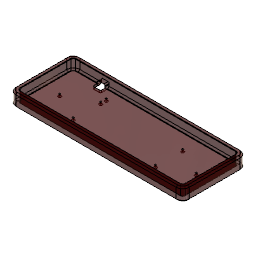
PlanckHiProCase (Autodesk Fusion 360 design; units mm, degrees)
part number: 2025-12-26-20-35-43-522
Autodesk Fusion 360 part; units mm, degrees
ref_plane "WorkPlane1" through (0, 0, -6) normal (0, 0, 1) x (1, 0, 0)
ref_plane "WorkPlane2" through (0, 0, -5) normal (0, 0, 1) x (1, 0, 0)
other "Base Mesh Feature2"
sketch "Floor" plane through (0, 0, -5) normal (0, 0, 1) x (1, 0, 0)
  circle A0 centre (-95, -0.0001) radius 1.0986
  circle A1 centre (-56.999, 27.0014) radius 0.9987
  circle A2 centre (-57, 18.9999) radius 1.0986
  circle A3 centre (-57, -19) radius 1.0985
  circle A4 centre (57, -19) radius 1.0985
  circle A5 centre (57, 18.9999) radius 1.0986
  circle A6 centre (95, -0.0001) radius 1.0986
  line L0 (-81.249, 50.7868) -> (-81.249, 32.4014)
  line L1 (-81.249, 32.4014) -> (-70.749, 32.4014)
  line L2 (-70.749, 32.4014) -> (-70.749, 50.7879)
  line L3 (-81.249, 50.7868) -> (-70.749, 50.7879)
  dimension "d10" = 10.5
  dimension "d21" = 5.4
  dimension "d22" = 13.75
  constraint horizontal L1
  constraint vertical L0
  constraint vertical L2
  constraint coincident L0.end L1.start
  constraint coincident L1.end L2.start
  measures "d10" distance of L0 L2
  measures "d21" distance of A1.centre L1
  measures "d22" distance of A1.centre L2
other "MeshSection1"
sketch "Walls" plane through (0, 0, -6) normal (0, 0, 1) x (1, 0, 0)
  line L0 (111.325, 38.5) -> (-111.325, 38.5)
  arc A0 (114.5, 35.325) -> (111.325, 38.5) centre (111.325, 35.325) ccw
  line L1 (114.5, -35.325) -> (114.5, 35.325)
  arc A1 (111.325, -38.5) -> (114.5, -35.325) centre (111.325, -35.325) ccw
  line L2 (-111.325, -38.5) -> (111.325, -38.5)
  arc A2 (-114.5, -35.325) -> (-111.325, -38.5) centre (-111.325, -35.325) ccw
  line L3 (-114.5, 35.325) -> (-114.5, -35.325)
  arc A3 (-111.325, 38.5) -> (-114.5, 35.325) centre (-111.325, 35.325) ccw
  line L4 (-120.5, 35.325) -> (-120.5, -35.325)
  arc A4 (-120.5, -35.325) -> (-111.325, -44.5) centre (-111.325, -35.325) ccw
  line L5 (-111.325, -44.5) -> (111.325, -44.5)
  arc A5 (111.325, -44.5) -> (120.5, -35.325) centre (111.325, -35.325) ccw
  line L6 (120.5, -35.325) -> (120.5, 35.325)
  arc A6 (120.5, 35.325) -> (111.325, 44.5) centre (111.325, 35.325) ccw
  line L7 (111.325, 44.5) -> (-111.325, 44.5)
  arc A7 (-111.325, 44.5) -> (-120.5, 35.325) centre (-111.325, 35.325) ccw
  dimension "d23" = 38.5
  dimension "d24" = 38.5
  dimension "d25" = 114.5
  dimension "d26" = 114.5
  dimension "d28" = 3.175
  dimension "d29" = 6
  constraint horizontal L2
  constraint horizontal L0
  constraint tangent L2 A2
  constraint tangent A1 L2
  constraint tangent L0 A0
  constraint tangent L0 A3
  constraint tangent A2 L3
  constraint vertical L3
  constraint vertical L1
  constraint tangent L1 A1
  constraint tangent A0 L1
  constraint tangent L3 A3
  constraint coincident L3.start A3.end
  constraint equal A2 A3
  constraint equal A1 A3
  constraint equal A0 A3
  measures "d23" distance of origin L0
  measures "d24" distance of origin L2
  measures "d25" distance of origin L3
  measures "d26" distance of origin L1
  measures "d28" radius of A3
other "MeshSection2"
ref_plane "WorkPlane3" through (0, 38.5, 0) normal (0, 1, 0) x (0, 0, 1)
sketch "BackCutout" plane through (0, 38.5, 0) normal (0, 1, 0) x (-1, 0, 0)
  line L0 (70.75, -1.9309) -> (70.75, -14.816)
  line L1 (81.25, -1.9309) -> (70.75, -1.9309)
  line L2 (70.75, -14.816) -> (81.25, -14.816)
  line L3 (115.5, -9.0707) -> (70.75, -9.0709) construction
  line L4 (-115.5, -9.0698) -> (70.75, -9.0709) construction
  line L5 (81.25, -1.9309) -> (81.25, -14.816)
  point P0 (76, -1.9309)
  dimension "d37" = 7.14
  dimension "d39" = 5.25
  dimension "d40" = 5.25
  constraint horizontal L1
  constraint vertical L0
  constraint midpoint L1 P0
  constraint horizontal L2
  constraint vertical L5
  constraint coincident L1.start L5.start
  constraint coincident L0.start L1.end
  measures "d37" distance of P0 L3
  measures "d39" distance of P0 L5
  measures "d40" distance of L0 P0
other "MeshSection3"
extrude "Extrude1" add sketch "Walls" against normal blind 3 contours L0 A0 L1 A1 L2 A2 L3 A3 | L4 A4 L5 A5 L6 A6 L7 A7
extrude "Extrude2" add sketch "Walls" along normal blind 15
extrude "CutDown" cut sketch "Floor" against normal through all contours L0 L1 L2 L3
extrude "CutBack" cut sketch "BackCutout" along normal through all
chamfer "Chamfer1" distance 0.5 angle 45 8 edges at (-113.5701, 37.5701, 9) (0, 38.5, 9) (113.5701, 37.5701, 9) (114.5, 0, 9) (113.5701, -37.5701, 9) (0, -38.5, 9) (-113.5701, -37.5701, 9) (-114.5, 0, 9)
chamfer "Chamfer1" distance 2 angle 45 8 edges at (-120.5, 0, 9) (-117.8127, -41.8127, 9) (0, -44.5, 9) (117.8127, -41.8127, 9) (120.5, 0, 9) (117.8127, 41.8127, 9) (0, 44.5, 9) (-117.8127, 41.8127, 9)
chamfer "Chamfer1" distance 2 angle 45 9 edges at (-96.287, 44.5, -9) (20.288, 44.5, -9) (117.8127, 41.8127, -9) (120.5, 0, -9) (117.8127, -41.8127, -9) (0, -44.5, -9) (-117.8127, -41.8127, -9) (-120.5, 0, -9) (-117.8127, 41.8127, -9)
fillet "Fillet2" radius 1.5875 2 edges at (-81.249, 32.4014, -7.5) (-70.749, 32.4014, -7.5)
fillet "Fillet2" radius 1.5875 2 edges at (-81.25, 41.5, -1.9309) (-70.75, 41.5, -1.9309)
sketch "Holes" plane through (0, 0, -9) normal (0, 0, -1) x (1, 0, 0)
  line L0 (-81.249, -38.5) -> (-81.249, -33.9889)
  line L1 (-79.6615, -32.4014) -> (-72.3365, -32.4014)
  line L2 (-70.749, -33.9889) -> (-70.749, -42.5)
  line L3 (-81.25, -38.5) -> (-81.249, -38.5)
  line L4 (-81.25, -42.5) -> (-81.25, -38.5)
  arc A0 (-79.6615, -32.4014) -> (-81.249, -33.9889) centre (-79.6615, -33.9889) ccw
  arc A1 (-70.749, -33.9889) -> (-72.3365, -32.4014) centre (-72.3365, -33.9889) ccw
  line L5 (-70.749, -42.5) -> (111.325, -42.5)
  arc A2 (111.325, -42.5) -> (118.5, -35.325) centre (111.325, -35.325) ccw
  line L6 (118.5, -35.325) -> (118.5, 35.325)
  arc A3 (118.5, 35.325) -> (111.325, 42.5) centre (111.325, 35.325) ccw
  line L7 (111.325, 42.5) -> (-111.325, 42.5)
  arc A4 (-111.325, 42.5) -> (-118.5, 35.325) centre (-111.325, 35.325) ccw
  line L8 (-118.5, 35.325) -> (-118.5, -35.325)
  arc A5 (-118.5, -35.325) -> (-111.325, -42.5) centre (-111.325, -35.325) ccw
  line L9 (-111.325, -42.5) -> (-81.25, -42.5)
  point P0 (57, -18.9999)
  point P1 (95, 0.0001)
  point P2 (57, 19)
  point P3 (-57, 19)
  point P4 (-95, 0.0001)
  point P5 (-57, -18.9999)
  point P6 (-56.999, -27.0014)
hole "Hole1" at (57, -19, -9) at (57, 18.9999, -9) at (95, -0.0001, -9) at (-57, 18.9999, -9) at (-57, -19, -9) at (-95, -0.0001, -9) at (-56.999, 27.0014, -9) direction (0, 0, 1) diameter 2.2 end through all countersink diameter 4 countersink angle 90
equation "d26 = d25"
equation "d28 = 1 in / 8"
equation "smallFillet = 1 in / 16"
equation "d40 = d39"
equation "d42 = smallFillet"
equation "d44 = smallFillet"
